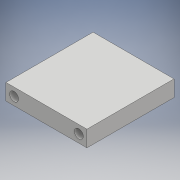
# Autodesk Inventor part: support_moteur
Saved by Autodesk Inventor 2017 (Build 210142000, 142)
## iProperties
Part Number: support_moteur
Material: Générique
Document SubType Name: Modeling
Designer: ElsaT
Density: 1 g/cm^3
Appearance: Par défaut
Author: ElsaT
## iProperties of the stored document support_moteur_Impression 3D.ipt
Part Number: support_moteur_Impression 3D
Material: Générique
Document SubType Name: Modeling
Designer: ElsaT
Density: 1 g/cm^3
Appearance: Par défaut
Author: ElsaT
Autodesk Inventor part; units mm, degrees
ref_plane "YZ Plane" through (0, 0, 0) normal (1, 0, 0) x (0, 1, 0)
ref_plane "XZ Plane" through (0, 0, 0) normal (0, 1, 0) x (-1, 0, 0)
ref_plane "XY Plane" through (0, 0, 0) normal (0, 0, 1) x (1, 0, 0)
sketch "Esquisse1" plane through (0, 0, 0) normal (0, 1, 0) x (-1, 0, 0)
  line L0 (-25, 5) -> (25, 5)
  line L1 (25, 5) -> (25, -5)
  line L2 (25, -5) -> (-25, -5)
  line L3 (-25, -5) -> (-25, 5)
  line L4 (-25, 5) -> (25, -5) construction
  line L5 (25, 5) -> (-25, -5) construction
  point P0 (0, 0)
  dimension "d0" = 50
  dimension "d1" = 10
  constraints: 12 end point, 2 midpoint, 2 parallel, 1 horizontal, 1 perpendicular
  measures "d0" distance of L1.end L2.end
  measures "d1" distance of L0.end L1.end
extrude "Extrusion1" add sketch "Esquisse1" along normal blind 53.8
sketch "Esquisse2" plane through (0, 53.8, 0) normal (0, 1, 0) x (1, 0, 0)
  circle A0 centre (-20, 0) radius 2.75
  circle A1 centre (20, 0) radius 2.75
  line L0 (-25, -5) -> (25, -5) projected
  line L1 (-25, 5) -> (-25, -5) projected
  line L2 (25, -5) -> (25, 5) projected
  point P0 (0, 0)
  dimension "d4" = 5.5
  dimension "d5" = 5.5
  dimension "d6" = 5
  dimension "d7" = 5
  dimension "d8" = 5
  dimension "d9" = 5
  constraints: 2 centre point
  measures "d4" diameter of A0
  measures "d5" diameter of A1
  measures "d6" distance from line of L0 A0.centre
  measures "d7" distance from line of L0 A1.centre
  measures "d8" distance from line of L1 A0.centre
  measures "d9" distance from line of L2 A1.centre
extrude "Extrusion2" cut sketch "Esquisse2" against normal blind 53.8
